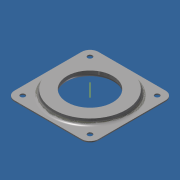
# Autodesk Inventor part: 70mmkugellager
Saved by Autodesk Inventor 2014 SP2 (Build 180246200, 246)
## iProperties
Created: 2015-01-20
Part Number: 70mmkugellager
Material: Stahl, galvanisiert
Document SubType Name: Modeling
Designer: 4ndreas
Density: 7.85 g/cm^3
Appearance: Galvanisiert
Author: 4ndreas
Autodesk Inventor part; units mm, degrees
ref_plane "YZ Plane" through (0, 0, 0) normal (1, 0, 0) x (0, 1, 0)
ref_plane "XZ Plane" through (0, 0, 0) normal (0, 1, 0) x (-1, 0, 0)
ref_plane "XY Plane" through (0, 0, 0) normal (0, 0, 1) x (1, 0, 0)
sketch "Skizze1" plane through (0, 0, 0) normal (0, 0, 1) x (1, 0, 0)
  line L0 (-35, 35) -> (35, 35)
  line L1 (35, 35) -> (35, -35)
  line L2 (35, -35) -> (-35, -35)
  line L3 (-35, -35) -> (-35, 35)
  circle A0 centre (0, 0) radius 35
  circle A1 centre (0, 0) radius 19
  dimension "d0" = 70
  dimension "d1" = 38
  constraints: 8 end point, 4 tangent, 2 centre point, 2 coincident, 2 parallel, 1 horizontal, 1 perpendicular
  measures "d0" distance between parallel lines of L2 L0
  measures "d1" diameter of A1
extrude "Extrusion1" add sketch "Skizze1" along normal blind 0.9
fillet "Rundung1" radius 7 4 edges at (-35, -35, 0.45) (35, -35, 0.45) (-35, 35, 0.45) (35, 35, 0.45)
sketch "Skizze2" plane through (0, 0, 0.9) normal (0, 0, 1) x (1, 0, 0)
  arc A0 (35, 28) -> (28, 35) centre (28, 28) ccw projected
  arc A1 (-28, 35) -> (-35, 28) centre (-28, 28) ccw projected
  arc A2 (-35, -28) -> (-28, -35) centre (-28, -28) ccw projected
  arc A3 (28, -35) -> (35, -28) centre (28, -28) ccw projected
  dimension "d16" = 56
  measures "d16" distance of A1.centre A0.centre
hole "Bohrung1" at (-28, -28, 0.9) at (28, -28, 0.9) at (28, 28, 0.9) at (-28, 28, 0.9) direction (0, 0, -1) diameter 4 depth 8 tip angle 118
sketch "Skizze3" plane through (0, 0, 0.9) normal (0, 0, 1) x (1, 0, 0)
  circle A0 centre (0, 0) radius 19 projected
  circle A1 centre (0, 0) radius 30
  dimension "d12" = 60
  constraints: 1 centre point, 1 coincident
  measures "d12" diameter of A1
extrude "Extrusion2" add sketch "Skizze3" along normal blind 4.6
fillet "Rundung2" radius 3 2 edges at (-19, 0, 0) (-30, 0, 0.9)
